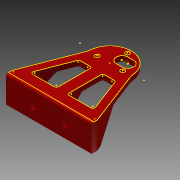
# Autodesk Inventor part: motor holder
Saved by Autodesk Inventor 2013 (Build 170138000, 138)
## iProperties
Created: 2015-01-06
Part Number: motor holder
Material: Generic
Document SubType Name: Modeling
Designer: Nico
Density: 1 g/cm^3
Author: Nico
Autodesk Inventor part; units mm, degrees
ref_plane "YZ Plane" through (0, 0, 0) normal (1, 0, 0) x (0, 1, 0)
ref_plane "XZ Plane" through (0, 0, 0) normal (0, 1, 0) x (-1, 0, 0)
ref_plane "XY Plane" through (0, 0, 0) normal (0, 0, 1) x (1, 0, 0)
sketch "Sketch1" plane through (0, 0, 0) normal (0, 0, 1) x (1, 0, 0)
  arc A0 (19.9536, 1.3617) -> (-19.9536, 1.3617) centre (0, 0) ccw
  circle A1 centre (-12, 0) radius 2
  circle A2 centre (12, 0) radius 2
  circle A3 centre (0, 16.5) radius 2
  line L0 (9, 2.7139) -> (3, 2.7139)
  line L1 (-2, 7.7139) -> (-2, 8.4978)
  line L2 (3, 13.4978) -> (9, 13.4978)
  line L3 (14, 8.4978) -> (14, 7.7139)
  arc A4 (14, 8.4978) -> (9, 13.4978) centre (9, 8.4978) ccw
  arc A5 (9, 2.7139) -> (14, 7.7139) centre (9, 7.7139) ccw
  arc A6 (-2, 7.7139) -> (3, 2.7139) centre (3, 7.7139) ccw
  arc A7 (3, 13.4978) -> (-2, 8.4978) centre (3, 8.4978) ccw
  line L4 (20, -51.8414) -> (-20, -51.8414)
  line L5 (-20.6006, -1.5568) -> (-40, -51.8414)
  line L6 (-20, -51.8414) -> (-40, -51.8414)
  line L7 (20.6006, -1.5568) -> (40, -51.8414)
  line L8 (40, -51.8414) -> (20, -51.8414)
  arc A8 (-20.6006, -1.5568) -> (-19.9536, 1.3617) centre (-29.9304, 2.0425) ccw
  arc A9 (19.9536, 1.3617) -> (20.6006, -1.5568) centre (29.9304, 2.0425) ccw
  point P0 (-20, 0)
  point P1 (20, 0)
  dimension "d3" = 40
  dimension "d4" = 4
  dimension "d5" = 4
  dimension "d6" = 4
  dimension "d7" = 12
  dimension "d8" = 12
  dimension "d9" = 16.5
  dimension "d10" = 5
  dimension "d13" = 10
  constraints: 18 end point, 16 point on circle, 12 tangent, 10 centre point, 4 equal radius, 3 equal length, 2 point on line, 1 horizontal, 1 perpendicular
  measures "d3" diameter of A0
  measures "d4" diameter of A1
  measures "d5" diameter of A3
  measures "d6" diameter of A2
  measures "d7" distance of point (0, 0) A2.centre
  measures "d8" distance of A1.centre point (0, 0)
  measures "d9" distance of point (0, 0) A3.centre
  measures "d10" radius of A4
  measures "d13" radius of A8
extrude "Extrusion1" add sketch "Sketch1" along normal blind 5
sketch "Sketch4" plane through (-40, -51.8414, 0) normal (0, -1, 0) x (1, 0, 0)
  line L0 (0, 5) -> (80, 5)
  line L1 (80, 5) -> (80, -20)
  line L2 (80, -20) -> (0, -20)
  line L3 (0, -20) -> (0, 5)
  point P0 (40, 0)
  dimension "d40" = 25
  constraints: 8 end point, 2 parallel, 1 horizontal, 1 perpendicular
  measures "d40" distance between parallel lines of L2 L0
extrude "Extrusion2" add sketch "Sketch4" along normal blind 5
fillet "Fillet1" radius 2 1 edges at (0, -56.8414, 5)
sketch "Sketch5" plane through (0, 0, 0) normal (0, 0, -1) x (-1, 0, 0)
  line L0 (-40, -51.8414) -> (40, -51.8414) projected
  line L1 (40, -51.8414) -> (20.6006, -1.5568) projected
  arc A0 (19.9536, 1.3617) -> (-19.9536, 1.3617) centre (0, 0) ccw projected
  line L2 (-20.6006, -1.5568) -> (-40, -51.8414) projected
  line L3 (-30, -45.0013) -> (-17.1567, -11.7105)
  line L4 (-17.1567, -11.7105) -> (-5, -11.7105)
  line L5 (-5, -11.7105) -> (-5, -45.0013)
  line L6 (-5, -45.0013) -> (-30, -45.0013)
  line L7 (5, -11.7105) -> (17.1567, -11.7105)
  line L8 (17.1567, -11.7105) -> (30, -45.0013)
  line L9 (30, -45.0013) -> (5, -45.0013)
  line L10 (5, -45.0013) -> (5, -13.4701)
  line L11 (5, -13.4701) -> (5, -11.7105)
  line L12 (40, -56.8414) -> (-40, -56.8414) projected
  dimension "d45" = 5
  dimension "d46" = 5
  dimension "d47" = 25
  dimension "d48" = 25
  dimension "d49" = 12.1567
  dimension "d87" = 33.2908
  dimension "d88" = 11.8401
  constraints: 18 end point, 5 parallel, 3 perpendicular, 1 collinear
  measures "d45" distance from line of L10 A0.centre
  measures "d46" distance from line of L5 A0.centre
  measures "d47" distance of L5.end L3.start
  measures "d48" distance of L8.end L9.end
  measures "d49" distance of L3.end L4.end
  measures "d87" distance of L4.end L5.end
  measures "d88" distance between parallel lines of L12 L6
extrude "Extrusion3" cut sketch "Sketch5" against normal blind 5
sketch "Sketch6" plane through (0, 0, 0) normal (0, 0, -1) x (-1, 0, 0)
  line L0 (-40, -51.8414) -> (40, -51.8414) projected
  arc A0 (19.9536, 1.3617) -> (-19.9536, 1.3617) centre (0, 0) ccw projected
  line L1 (-3, -51.8414) -> (3, -51.8414)
  line L2 (3, -51.8414) -> (3, -26.8414)
  line L3 (3, -26.8414) -> (-3, -26.8414)
  line L4 (-3, -26.8414) -> (-3, -51.8414)
  dimension "d52" = 25
  dimension "d54" = 3
  dimension "d55" = 3
  constraints: 8 end point, 2 parallel, 1 horizontal, 1 perpendicular, 1 point on line
  measures "d52" distance of L3.end L1.start
  measures "d54" distance from line of L4 A0.centre
  measures "d55" distance from line of L2 A0.centre
extrude "Extrusion4" add sketch "Sketch6" along normal blind 20
chamfer "Chamfer1" distance 20 distance2 20 1 edges at (0, -26.8414, -20) measured on face at (-1, -55.1748, -20)
sketch "Sketch7" plane through (0, 0, 0) normal (0, 0, -1) x (-1, 0, 0)
  line L0 (-3, -26.8414) -> (3, -26.8414) projected
  line L1 (3, -51.8414) -> (40, -51.8414) projected
  line L2 (40, -51.8414) -> (20.6006, -1.5568) projected
  line L3 (-20.6006, -1.5568) -> (-40, -51.8414) projected
  line L4 (-40, -51.8414) -> (-3, -51.8414) projected
  line L5 (17.1567, -11.7105) -> (30, -45.0013) projected
  line L6 (-30, -45.0013) -> (-17.1567, -11.7105) projected
  line L7 (-5, -11.7105) -> (-5, -45.0013) projected
  line L8 (-40, -51.8414) -> (-30.3003, -26.6991)
  line L9 (-30.3003, -26.6991) -> (-22.9392, -26.6991)
  line L10 (-22.9392, -26.6991) -> (-32.6389, -51.8414)
  line L11 (-32.6389, -51.8414) -> (-40, -51.8414)
  line L12 (22.9392, -26.6991) -> (30.3003, -26.6991)
  line L13 (30.3003, -26.6991) -> (40, -51.8414)
  line L14 (22.9392, -26.6991) -> (32.6389, -51.8414)
  line L15 (32.6389, -51.8414) -> (40, -51.8414)
  line L16 (40, -51.8414) -> (32.6389, -51.8414)
  dimension "d61" = 0.1423
  constraints: 18 end point, 6 point on line, 4 parallel, 2 collinear, 2 midpoint, 1 perpendicular
  measures "d61" distance between parallel lines of L0 L9
extrude "Extrusion5" add sketch "Sketch7" along normal blind 20
chamfer "Chamfer2" distance 20 distance2 20 1 edges at (-26.6197, -26.6991, -20)
chamfer "Chamfer3" distance 20 distance2 20 1 edges at (26.6197, -26.6991, -20)
sketch "Sketch8" plane through (-40, -51.8414, 0) normal (0, 1, 0) x (1, 0, 0)
  line L0 (43, 20) -> (72.6389, 20) projected
  line L1 (0, 20) -> (0, -5) projected
  line L2 (80, 20) -> (80, -5) projected
  line L3 (7.3611, 20) -> (37, 20) projected
  point P0 (40, 0)
  point P1 (25, 10)
  point P2 (55, 10)
  dimension "d70" = 25
  dimension "d71" = 25
  dimension "d72" = 10
  dimension "d73" = 10
  measures "d70" distance from line of point (25, 10) L1
  measures "d71" distance from line of point (55, 10) L2
  measures "d72" distance from line of point (55, 10) L0
  measures "d73" distance from line of point (25, 10) L3
hole "Hole1" at (-15, -51.8414, -10) at (15, -51.8414, -10) direction (0, -1, 0) diameter 4 end through all
fillet "Fillet2" radius 2 8 edges at (30, -45.0013, 2.5) (-5, -45.0013, 2.5) (-30, -45.0013, 2.5) (5, -45.0013, 2.5) (-17.1567, -11.7105, 2.5) (5, -11.7105, 2.5) (17.1567, -11.7105, 2.5) (-5, -11.7105, 2.5)
fillet "Fillet3" radius 2 1 edges at (-40, -51.8414, -7.5)
fillet "Fillet4" radius 2 1 edges at (40, -51.8414, -7.5)
fillet "Fillet5" radius 2 2 edges at (-32.6389, -51.8414, -10) (32.6389, -51.8414, -10)
fillet "Fillet6" radius 2 8 edges at (31.3728, -50.9729, 0) (29.4753, -43.6414, 0) (16.3618, -51.8414, 0) (-31.3728, -50.9729, 0) (-29.4753, -43.6414, 0) (-16.3618, -51.8414, 0) (-3, -51.8414, -10) (3, -51.8414, -10)
fillet "Fillet7" radius 2 4 edges at (-26.6197, -26.6991, 0) (26.6197, -26.6991, 0) (34.3356, -46.6991, -20) (-34.3356, -46.6991, -20)
sketch "Sketch9" plane through (0, 0, 5) normal (0, 0, 1) x (1, 0, 0)
  arc A0 (40, -52.2139) -> (39.866, -51.494) centre (38, -52.2139) ccw projected
  line L0 (39.866, -51.494) -> (20.6006, -1.5568) projected
  arc A1 (19.9536, 1.3617) -> (20.6006, -1.5568) centre (29.9304, 2.0425) ccw projected
  arc A2 (19.9536, 1.3617) -> (-19.9536, 1.3617) centre (0, 0) ccw projected
  arc A3 (-20.6006, -1.5568) -> (-19.9536, 1.3617) centre (-29.9304, 2.0425) ccw projected
  line L1 (-20.6006, -1.5568) -> (-39.866, -51.494) projected
  arc A4 (-39.866, -51.494) -> (-40, -52.2139) centre (-38, -52.2139) ccw projected
  line L2 (-40, -52.2139) -> (-40, -54.8414) projected
  line L3 (40, -54.8414) -> (-40, -54.8414) projected
  line L4 (40, -52.2139) -> (40, -54.8414) projected
  line L5 (27.0847, -45.0013) -> (7, -45.0013) projected
  arc A5 (5, -43.0013) -> (7, -45.0013) centre (7, -43.0013) ccw projected
  line L6 (5, -43.0013) -> (5, -13.7105) projected
  arc A6 (7, -11.7105) -> (5, -13.7105) centre (7, -13.7105) ccw projected
  line L7 (7, -11.7105) -> (15.7846, -11.7105) projected
  arc A7 (17.6505, -12.9907) -> (15.7846, -11.7105) centre (15.7846, -13.7105) ccw projected
  line L8 (17.6505, -12.9907) -> (28.9507, -42.2815) projected
  arc A8 (27.0847, -45.0013) -> (28.9507, -42.2815) centre (27.0847, -43.0013) ccw projected
  line L9 (-5, -13.7105) -> (-5, -43.0013) projected
  arc A9 (-7, -45.0013) -> (-5, -43.0013) centre (-7, -43.0013) ccw projected
  line L10 (-7, -45.0013) -> (-27.0847, -45.0013) projected
  arc A10 (-28.9507, -42.2815) -> (-27.0847, -45.0013) centre (-27.0847, -43.0013) ccw projected
  line L11 (-28.9507, -42.2815) -> (-17.6505, -12.9907) projected
  arc A11 (-15.7846, -11.7105) -> (-17.6505, -12.9907) centre (-15.7846, -13.7105) ccw projected
  line L12 (-15.7846, -11.7105) -> (-7, -11.7105) projected
  arc A12 (-5, -13.7105) -> (-7, -11.7105) centre (-7, -13.7105) ccw projected
  arc A13 (9, 2.7139) -> (14, 7.7139) centre (9, 7.7139) ccw projected
  line L13 (9, 2.7139) -> (3, 2.7139) projected
  arc A14 (-2, 7.7139) -> (3, 2.7139) centre (3, 7.7139) ccw projected
  line L14 (-2, 7.7139) -> (-2, 8.4978) projected
  arc A15 (3, 13.4978) -> (-2, 8.4978) centre (3, 8.4978) ccw projected
  line L15 (3, 13.4978) -> (9, 13.4978) projected
  arc A16 (14, 8.4978) -> (9, 13.4978) centre (9, 8.4978) ccw projected
  line L16 (14, 8.4978) -> (14, 7.7139) projected
  circle A17 centre (0, 16.5) radius 2 projected
  circle A18 centre (12, 0) radius 2 projected
  circle A19 centre (-12, 0) radius 2 projected
  point P0 (6, 8.4978)
chamfer "Chamfer4" distance 1 angle 45 1 edges at (-14, 0, 5)
chamfer "Chamfer5" distance 1 angle 45 1 edges at (-2, 16.5, 5)
chamfer "Chamfer6" distance 1 angle 45 1 edges at (10, 0, 5)
equation "\"BendRadius\" = Thickness"
equation "\"BendReliefWidth\" = Thickness"
equation "\"BendReliefDepth\" = 0.5 * Thickness"
equation "\"CornerReliefSize\" = 4 * Thickness"
equation "\"MinimumRemnant\" = 2 * Thickness"
equation "\"TransitionRadius\" = BendRadius"
equation "\"JacobiRadiusSize\" = BendRadius"
equation "\"GapSize\" = Thickness"
equation "\"d14\" = BendRadius"
equation "\"Thickness\" = 3"
body "Solid2"
